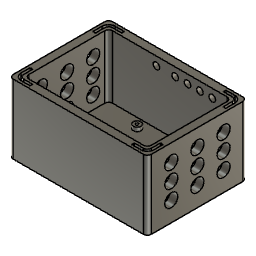
boitier_raspi (Autodesk Fusion 360 design; units mm, degrees)
Autodesk Fusion 360 part; units mm, degrees
sketch "Esquisse1" plane through (0, 0, 0) normal (0, 0, 1) x (1, 0, 0)
  line L0 (3.5419, 0) -> (103.2419, 0)
  line L1 (106.2419, 3) -> (106.2419, 73)
  line L2 (0.5419, 73) -> (0.5419, 3)
  line L3 (9.5419, 6) -> (97.2419, 6)
  line L4 (100.2419, 9) -> (100.2419, 67)
  line L5 (97.2419, 70) -> (9.5419, 70)
  line L6 (6.5419, 67) -> (6.5419, 9)
  arc A0 (100.2419, 67) -> (97.2419, 70) centre (97.2419, 67) ccw
  arc A1 (97.2419, 6) -> (100.2419, 9) centre (97.2419, 9) ccw
  arc A2 (6.5419, 9) -> (9.5419, 6) centre (9.5419, 9) ccw
  arc A3 (9.5419, 70) -> (6.5419, 67) centre (9.5419, 67) ccw
  circle A4 centre (93.7419, 62.62) radius 3
  circle A5 centre (93.7419, 62.62) radius 1.125
  circle A6 centre (93.7419, 13.62) radius 3
  circle A7 centre (93.7419, 13.62) radius 1.125
  circle A8 centre (35.7419, 13.62) radius 1.125
  circle A9 centre (35.7419, 13.62) radius 3
  circle A10 centre (35.7419, 62.62) radius 3
  circle A11 centre (35.7419, 62.62) radius 1.125
  line L7 (103.2419, 76) -> (3.5419, 76)
  arc A12 (106.2419, 73) -> (103.2419, 76) centre (103.2419, 73) ccw
  arc A13 (3.5419, 76) -> (0.5419, 73) centre (3.5419, 73) ccw
  arc A14 (0.5419, 3) -> (3.5419, 0) centre (3.5419, 3) ccw
  arc A15 (103.2419, 0) -> (106.2419, 3) centre (103.2419, 3) ccw
  line L8 (86.6419, 76) -> (86.6419, 70)
  point P0 (6.5419, 6)
  point P1 (100.2419, 6)
  point P2 (6.5419, 70)
  dimension "d5" = 6
  dimension "d6" = 6
  dimension "d7" = 3
  dimension "d8" = 3
  dimension "d9" = 3
  dimension "d10" = 3
  dimension "d34" = 6
  dimension "d37" = 2.25
  dimension "d38" = 6
  dimension "d39" = 2.25
  dimension "d40" = 6
  dimension "d41" = 2.25
  dimension "d42" = 58
  dimension "d47" = 6
  dimension "d48" = 2.25
  dimension "d52" = 6
  dimension "d77" = 64
  dimension "d80" = 6
  dimension "d85" = 7.62
  dimension "d86" = 6.5
  dimension "d88" = 7.62
  dimension "d89" = 58
  dimension "d90" = 49
  dimension "d93" = 6.5
  dimension "d94" = 49
  dimension "d101" = 3
  dimension "d102" = 3
  dimension "d103" = 3
  dimension "d104" = 3
  dimension "d105" = 7.1
  dimension "d178" = 76
  dimension "d179" = 105.7
  dimension "d223" = 29.2
  dimension "d260" = 7.38
  dimension "d263" = 13.38
  constraint horizontal L0
  constraint vertical L1
  constraint vertical L2
  constraint horizontal L3
  constraint vertical L4
  constraint horizontal L5
  constraint tangent L4 A0
  constraint tangent L5 A0
  constraint coincident P1 L3
  constraint coincident P1 L4
  constraint tangent L3 A1
  constraint tangent L4 A1
  constraint coincident P0 L3
  constraint coincident P0 L6
  constraint tangent L3 A2
  constraint tangent L6 A2
  constraint coincident P2 L5
  constraint coincident P2 L6
  constraint tangent L5 A3
  constraint tangent L6 A3
  constraint concentric A4 A5
  constraint concentric A6 A7
  constraint concentric A8 A9
  constraint concentric A10 A11
  constraint perpendicular L2 L7
  constraint tangent L7 A12
  constraint tangent L1 A12
  constraint tangent L7 A13
  constraint tangent L2 A13
  constraint tangent L0 A14
  constraint tangent L2 A14
  constraint tangent L0 A15
  constraint tangent L1 A15
  constraint coincident L7 L8.start
  constraint coincident L5 L8.end
  constraint perpendicular L5 L8
  measures "d5" distance of L0 L3
  measures "d6" distance of L1 L4
  measures "d7" radius of A0
  measures "d8" radius of A1
  measures "d9" radius of A2
  measures "d10" radius of A3
  measures "d34" diameter of A4
  measures "d37" diameter of A5
  measures "d38" diameter of A6
  measures "d39" diameter of A7
  measures "d40" diameter of A9
  measures "d41" diameter of A8
  measures "d42" distance of A6.centre A8.centre
  measures "d47" diameter of A10
  measures "d48" diameter of A11
  measures "d52" distance of L5 L7
  measures "d77" distance of L3 L5
  measures "d80" distance of L2 L6
  measures "d85" distance of L3 A6.centre
  measures "d86" distance of L4 A6.centre
  measures "d88" distance of L3 A8.centre
  measures "d89" horizontal distance of A4.centre A10.centre
  measures "d90" distance of A8.centre A10.centre
  measures "d93" distance of L4 A4.centre
  measures "d94" distance of A4.centre A6.centre
  measures "d101" radius of A12
  measures "d102" radius of A13
  measures "d103" radius of A14
  measures "d104" radius of A15
  measures "d105" distance of A4.centre L8
  measures "d178" distance of L0 L7
  measures "d179" distance of L1 L2
  measures "d223" distance of L6 A10.centre
  measures "d260" distance of L5 A10.centre
  measures "d263" distance of A4.centre L7
extrude "Extrusion1" add sketch "Esquisse1" along normal blind 5 contours L3 L4 L5 L6 A0 A1 A2 A3 | A4 | A5 | A6 | A7 | A8 | A9 | A10 | A11
extrude "Extrusion2" add sketch "Esquisse1" along normal blind 8 contours A4 | A6 | A9 | A10
extrude "Extrusion3" add sketch "Esquisse1" along normal blind 53 contours L0 L1 L2 L7 A12 A13 A14 A15
sketch "Esquisse4" plane through (0, 76, 0) normal (0, 1, 0) x (-1, 0, 0)
  line L0 (-103.2419, 0) -> (-3.5419, 0)
  line L1 (-3.5419, 0) -> (-3.5419, 53)
  line L2 (-3.5419, 53) -> (-103.2419, 53)
  line L3 (-103.2419, 53) -> (-103.2419, 0)
  line L4 (-86.7419, 0) -> (-86.7419, 10.8)
  line L5 (-81.2419, 7.3) -> (-92.2419, 7.3)
  line L6 (-92.2419, 7.3) -> (-92.2419, 14.3)
  line L7 (-92.2419, 14.3) -> (-81.2419, 14.3)
  line L8 (-81.2419, 14.3) -> (-81.2419, 7.3)
  line L9 (-81.2419, 7.3) -> (-92.2419, 14.3) construction
  line L10 (-92.2419, 7.3) -> (-81.2419, 14.3) construction
  line L11 (-91.1319, 49) -> (-39.1319, 49)
  line L12 (-39.1319, 49) -> (-39.1319, 44)
  line L13 (-39.1319, 44) -> (-91.1319, 44)
  line L14 (-91.1319, 44) -> (-91.1319, 49)
  line L15 (-106.2419, 0) -> (-106.2419, 53)
  line L16 (-83.3319, 44) -> (-88.3319, 44)
  line L17 (-88.3319, 44) -> (-88.3319, 49)
  line L18 (-88.3319, 49) -> (-83.3319, 49)
  line L19 (-83.3319, 49) -> (-83.3319, 44)
  line L20 (-83.3319, 44) -> (-88.3319, 49) construction
  line L21 (-88.3319, 44) -> (-83.3319, 49) construction
  line L22 (-73.8819, 44) -> (-78.8819, 44)
  line L23 (-78.8819, 44) -> (-78.8819, 49)
  line L24 (-78.8819, 49) -> (-73.8819, 49)
  line L25 (-73.8819, 49) -> (-73.8819, 44)
  line L26 (-73.8819, 44) -> (-78.8819, 49) construction
  line L27 (-78.8819, 44) -> (-73.8819, 49) construction
  line L28 (-64.4319, 44) -> (-69.4319, 44)
  line L29 (-69.4319, 44) -> (-69.4319, 49)
  line L30 (-69.4319, 49) -> (-64.4319, 49)
  line L31 (-64.4319, 49) -> (-64.4319, 44)
  line L32 (-64.4319, 44) -> (-69.4319, 49) construction
  line L33 (-69.4319, 44) -> (-64.4319, 49) construction
  line L34 (-54.9819, 44) -> (-59.9819, 44)
  line L35 (-59.9819, 44) -> (-59.9819, 49)
  line L36 (-59.9819, 49) -> (-54.9819, 49)
  line L37 (-54.9819, 49) -> (-54.9819, 44)
  line L38 (-54.9819, 44) -> (-59.9819, 49) construction
  line L39 (-59.9819, 44) -> (-54.9819, 49) construction
  line L40 (-40.6319, 44) -> (-45.6319, 44)
  line L41 (-45.6319, 44) -> (-45.6319, 49)
  line L42 (-45.6319, 49) -> (-40.6319, 49)
  line L43 (-40.6319, 49) -> (-40.6319, 44)
  line L44 (-40.6319, 44) -> (-45.6319, 49) construction
  line L45 (-45.6319, 44) -> (-40.6319, 49) construction
  circle A0 centre (-85.8319, 46.5) radius 2.5
  circle A1 centre (-76.3819, 46.5) radius 2.5
  circle A2 centre (-66.9319, 46.5) radius 2.5
  circle A3 centre (-57.4819, 46.5) radius 2.5
  circle A4 centre (-43.1319, 46.5) radius 2.5
  point P0 (-86.7419, 10.8)
  point P1 (-85.8319, 46.5)
  point P2 (-76.3819, 46.5)
  point P3 (-66.9319, 46.5)
  point P4 (-57.4819, 46.5)
  point P5 (-43.1319, 46.5)
  dimension "d106" = 16.5
  dimension "d107" = 10.8
  dimension "d108" = 11
  dimension "d109" = 7
  dimension "d188" = 5
  dimension "d189" = 15.11
  dimension "d190" = 52
  dimension "d225" = 5
  dimension "d226" = 5
  dimension "d227" = 5
  dimension "d228" = 5
  dimension "d229" = 5.3
  dimension "d230" = 14.75
  dimension "d231" = 5
  dimension "d232" = 5
  dimension "d233" = 5
  dimension "d234" = 5
  dimension "d235" = 24.2
  dimension "d236" = 33.65
  dimension "d237" = 5
  dimension "d238" = 5
  dimension "d239" = 48
  dimension "d264" = 4
  dimension "d265" = 4.45
  dimension "d266" = 4.45
  dimension "d267" = 4.45
  constraint coincident L0 L4.start
  constraint perpendicular L0 L4
  constraint horizontal L5
  constraint perpendicular L5 L6
  constraint parallel L5 L7
  constraint parallel L6 L8
  constraint coincident L9 P0
  constraint coincident L10 P0
  constraint coincident P0 L4.end
  constraint horizontal L11
  constraint vertical L12
  constraint horizontal L13
  constraint vertical L14
  constraint horizontal L16
  constraint perpendicular L16 L17
  constraint parallel L16 L18
  constraint parallel L17 L19
  constraint coincident L20 P1
  constraint coincident L21 P1
  constraint horizontal L22
  constraint perpendicular L22 L23
  constraint parallel L22 L24
  constraint parallel L23 L25
  constraint coincident L26 P2
  constraint coincident L27 P2
  constraint horizontal L28
  constraint perpendicular L28 L29
  constraint parallel L28 L30
  constraint parallel L29 L31
  constraint coincident L32 P3
  constraint coincident L33 P3
  constraint horizontal L34
  constraint perpendicular L34 L35
  constraint parallel L34 L36
  constraint parallel L35 L37
  constraint coincident L38 P4
  constraint coincident L39 P4
  constraint horizontal L40
  constraint perpendicular L40 L41
  constraint parallel L40 L42
  constraint parallel L41 L43
  constraint coincident L44 P5
  constraint coincident L45 P5
  constraint coincident P1 A0.centre
  constraint tangent L16 A0
  constraint coincident P2 A1.centre
  constraint tangent L22 A1
  constraint coincident P3 A2.centre
  constraint tangent L13 A2
  constraint coincident P4 A3.centre
  constraint tangent L34 A3
  constraint coincident P5 A4.centre
  constraint tangent L40 A4
  measures "d106" distance of L3 L4
  measures "d107" distance of L4.start P0
  measures "d108" distance of L6.end L7.end
  measures "d109" distance of L5.end L6.end
  measures "d188" distance of L11.end L12.end
  measures "d189" distance of L14 L15
  measures "d190" distance of L12 L14
  measures "d225" distance of L17.end L18.end
  measures "d226" distance of L16.end L17.end
  measures "d227" distance of L23.end L24.end
  measures "d228" distance of L22.end L23.end
  measures "d229" distance of L14 P1
  measures "d230" distance of L14 P2
  measures "d231" distance of L29.end L30.end
  measures "d232" distance of L28.end L29.end
  measures "d233" distance of L35.end L36.end
  measures "d234" distance of L34.end L35.end
  measures "d235" distance of L14 P3
  measures "d236" distance of L14 P4
  measures "d237" distance of L41.end L42.end
  measures "d238" distance of L40.end L41.end
  measures "d239" distance of L14 P5
  measures "d264" distance of L2 L11
  measures "d265" distance of L19 L23
  measures "d266" distance of L25 L29
  measures "d267" distance of L31 L35
extrude "Extrusion8" cut sketch "Esquisse4" against normal blind 6 contours L5 L6 L7 L8
sketch "Esquisse5" plane through (0, 0, 0) normal (0, 0, -1) x (1, 0, 0)
  arc A0 (106.2419, -3) -> (103.2419, 0) centre (103.2419, -3) ccw
  line L0 (103.2419, 0) -> (3.5419, 0)
  arc A1 (3.5419, 0) -> (0.5419, -3) centre (3.5419, -3) ccw
  line L1 (0.5419, -3) -> (0.5419, -73)
  arc A2 (0.5419, -73) -> (3.5419, -76) centre (3.5419, -73) ccw
  line L2 (3.5419, -76) -> (103.2419, -76)
  arc A3 (103.2419, -76) -> (106.2419, -73) centre (103.2419, -73) ccw
  line L3 (106.2419, -73) -> (106.2419, -3)
  line L4 (7.5419, -6) -> (17.5419, -6)
  line L5 (17.5419, -6) -> (17.5419, -16)
  line L6 (17.5419, -16) -> (7.5419, -16)
  line L7 (7.5419, -16) -> (7.5419, -6)
  line L8 (17.5419, -16) -> (12.5419, -16)
  line L9 (12.5419, -16) -> (12.5419, -11)
  line L10 (12.5419, -11) -> (17.5419, -11)
  line L11 (17.5419, -11) -> (17.5419, -16)
  line L12 (7.5419, -56) -> (17.5419, -56)
  line L13 (17.5419, -56) -> (17.5419, -66)
  line L14 (17.5419, -66) -> (7.5419, -66)
  line L15 (7.5419, -66) -> (7.5419, -56)
  line L16 (17.5419, -66) -> (12.5419, -66)
  line L17 (17.5419, -60) -> (17.5419, -66)
  line L18 (92.5419, -6) -> (82.5419, -6)
  line L19 (82.5419, -6) -> (82.5419, -16)
  line L20 (82.5419, -16) -> (92.5419, -16)
  line L21 (92.5419, -16) -> (92.5419, -6)
  line L22 (82.5419, -16) -> (87.5419, -16)
  line L23 (87.5419, -16) -> (87.5419, -11)
  line L24 (87.5419, -11) -> (82.5419, -11)
  line L25 (82.5419, -11) -> (82.5419, -16)
  line L26 (82.5419, -56) -> (92.5419, -56)
  line L27 (92.5419, -56) -> (92.5419, -66)
  line L28 (92.5419, -66) -> (82.5419, -66)
  line L29 (82.5419, -66) -> (82.5419, -56)
  line L30 (92.5419, -66) -> (87.5419, -66)
  line L31 (92.5419, -61) -> (92.5419, -66)
  line L32 (17.5419, -56) -> (12.5419, -56)
  line L33 (12.5419, -56) -> (12.5419, -61)
  line L34 (12.5419, -61) -> (17.5419, -61)
  line L35 (17.5419, -61) -> (17.5419, -56)
  line L36 (82.5419, -56) -> (87.5419, -56)
  line L37 (87.5419, -56) -> (87.5419, -61)
  line L38 (87.5419, -61) -> (82.5419, -61)
  line L39 (82.5419, -61) -> (82.5419, -56)
  dimension "d115" = 6
  dimension "d116" = 7
  dimension "d125" = 40
  dimension "d126" = 7
  dimension "d127" = 10
  dimension "d128" = 10
  dimension "d129" = 5
  dimension "d130" = 5
  dimension "d132" = 85
  dimension "d133" = 6
  dimension "d134" = 10
  dimension "d135" = 10
  dimension "d137" = 5
  dimension "d138" = 10
  dimension "d139" = 10
  dimension "d140" = 5
  dimension "d141" = 5
  dimension "d142" = 40
  dimension "d143" = 10
  dimension "d144" = 5
  dimension "d145" = 10
  dimension "d146" = 85
  dimension "d147" = 5
  dimension "d148" = 5
  dimension "d149" = 5
  dimension "d150" = 5
  constraint horizontal L4
  constraint vertical L5
  constraint horizontal L6
  constraint vertical L7
  constraint horizontal L8
  constraint vertical L9
  constraint horizontal L10
  constraint vertical L11
  constraint horizontal L12
  constraint vertical L13
  constraint horizontal L14
  constraint vertical L15
  constraint horizontal L16
  constraint vertical L17
  constraint horizontal L18
  constraint vertical L19
  constraint horizontal L20
  constraint vertical L21
  constraint horizontal L22
  constraint vertical L23
  constraint horizontal L24
  constraint vertical L25
  constraint horizontal L26
  constraint vertical L27
  constraint horizontal L28
  constraint vertical L29
  constraint horizontal L30
  constraint vertical L31
  constraint horizontal L32
  constraint vertical L33
  constraint horizontal L34
  constraint vertical L35
  constraint horizontal L36
  constraint vertical L37
  constraint horizontal L38
  constraint vertical L39
  measures "d115" distance of L0 L4
  measures "d116" distance of L1 L7
  measures "d125" distance of L6 L12
  measures "d126" distance of L1 L15
  measures "d127" distance of L18.start L18.end
  measures "d128" distance of L18.start L20.end
  measures "d129" distance of L19.end L22.end
  measures "d130" distance of L19.end L24.end
  measures "d132" distance of L7 L21
  measures "d133" distance of L0 L18
  measures "d134" distance of L5.end L6.end
  measures "d135" distance of L12.start L12.end
  measures "d137" distance of L9.end L10.end
  measures "d138" distance of L26.start L26.end
  measures "d139" distance of L26.start L28.end
  measures "d140" distance of L27.end L30.end
  measures "d141" distance of L27.end L31.start
  measures "d142" distance of L20 L26
  measures "d143" distance of L4.end L5.end
  measures "d144" distance of L8.end L9.end
  measures "d145" distance of L12.end L13.end
  measures "d146" distance of L15 L27
  measures "d147" distance of L12.end L32.end
  measures "d148" distance of L12.end L34.end
  measures "d149" distance of L26.start L36.end
  measures "d150" distance of L26.start L38.end
extrude "Extrusion9" cut sketch "Esquisse5" against normal blind 3 contours L4 L5 L6 L7 L9 L10 | L12 L13 L14 L15 L16 L17 L33 L34 | L18 L19 L20 L21 L23 L24 | L26 L27 L28 L29 L30 L31 L37 L38
sketch "Esquisse6" plane through (0, 0, 53) normal (0, 0, 1) x (-1, 0, 0)
  arc A0 (-9.5419, -70) -> (-6.5419, -67) centre (-9.5419, -67) ccw
  line L0 (-9.5419, -70) -> (-97.2419, -70)
  arc A1 (-100.2419, -67) -> (-97.2419, -70) centre (-97.2419, -67) ccw
  line L1 (-100.2419, -67) -> (-100.2419, -9)
  arc A2 (-97.2419, -6) -> (-100.2419, -9) centre (-97.2419, -9) ccw
  line L2 (-97.2419, -6) -> (-9.5419, -6)
  arc A3 (-6.5419, -9) -> (-9.5419, -6) centre (-9.5419, -9) ccw
  line L3 (-6.5419, -9) -> (-6.5419, -67)
  arc A4 (-103.2419, 0) -> (-106.2419, -3) centre (-103.2419, -3) ccw
  line L4 (-106.2419, -3) -> (-106.2419, -73)
  arc A5 (-106.2419, -73) -> (-103.2419, -76) centre (-103.2419, -73) ccw
  line L5 (-103.2419, -76) -> (-3.5419, -76)
  arc A6 (-3.5419, -76) -> (-0.5419, -73) centre (-3.5419, -73) ccw
  line L6 (-0.5419, -73) -> (-0.5419, -3)
  arc A7 (-0.5419, -3) -> (-3.5419, 0) centre (-3.5419, -3) ccw
  line L7 (-3.5419, 0) -> (-103.2419, 0)
  line L8 (-103.2419, -76) -> (-3.5419, -76)
  line L9 (-0.5419, -73) -> (-0.5419, -3)
  line L10 (-106.2419, -3) -> (-106.2419, -73)
  line L11 (-3.5419, 0) -> (-103.2419, 0)
  line L12 (-14.5419, -74) -> (-7.5419, -74)
  line L13 (-2.5419, -69) -> (-2.5419, -62)
  arc A8 (-7.5419, -74) -> (-2.5419, -69) centre (-7.5419, -69) ccw
  line L14 (-14.5419, -72) -> (-7.5419, -72)
  arc A9 (-7.5419, -72) -> (-4.5419, -69) centre (-7.5419, -69) ccw
  line L15 (-4.5419, -69) -> (-4.5419, -62)
  line L16 (-14.5419, -74) -> (-14.5419, -72)
  line L17 (-4.5419, -62) -> (-2.5419, -62)
  line L18 (-92.2419, -74) -> (-99.2419, -74)
  line L19 (-104.2419, -69) -> (-104.2419, -62)
  arc A10 (-104.2419, -69) -> (-99.2419, -74) centre (-99.2419, -69) ccw
  line L20 (-92.2419, -72) -> (-99.2419, -72)
  arc A11 (-102.2419, -69) -> (-99.2419, -72) centre (-99.2419, -69) ccw
  line L21 (-102.2419, -69) -> (-102.2419, -62)
  line L22 (-92.2419, -74) -> (-92.2419, -72)
  line L23 (-102.2419, -62) -> (-104.2419, -62)
  line L24 (-104.2419, -14) -> (-104.2419, -7)
  line L25 (-99.2419, -2) -> (-92.2419, -2)
  arc A12 (-99.2419, -2) -> (-104.2419, -7) centre (-99.2419, -7) ccw
  line L26 (-92.2419, -2) -> (-92.2419, -4)
  line L27 (-102.2419, -14) -> (-104.2419, -14)
  line L28 (-102.2419, -14) -> (-102.2419, -7)
  arc A13 (-99.2419, -4) -> (-102.2419, -7) centre (-99.2419, -7) ccw
  line L29 (-99.2419, -4) -> (-92.2419, -4)
  line L30 (-2.5419, -14) -> (-2.5419, -7)
  line L31 (-7.5419, -2) -> (-14.5419, -2)
  arc A14 (-2.5419, -7) -> (-7.5419, -2) centre (-7.5419, -7) ccw
  line L32 (-4.5419, -14) -> (-4.5419, -7)
  arc A15 (-4.5419, -7) -> (-7.5419, -4) centre (-7.5419, -7) ccw
  line L33 (-7.5419, -4) -> (-14.5419, -4)
  line L34 (-2.5419, -14) -> (-4.5419, -14)
  line L35 (-14.5419, -4) -> (-14.5419, -2)
  dimension "d277" = 5
  dimension "d278" = -2
  dimension "d279" = 2
  dimension "d280" = 2
  dimension "d281" = 12
  dimension "d282" = 12
  dimension "d283" = 5
  dimension "d284" = -2
  dimension "d285" = 12
  dimension "d286" = 12
  dimension "d287" = 5
  dimension "d288" = 2
  dimension "d289" = 2
  dimension "d290" = 2
  dimension "d291" = 2
  dimension "d292" = 2
  dimension "d293" = 12
  dimension "d294" = 12
  dimension "d295" = 2
  dimension "d296" = 2
  dimension "d297" = 5
  dimension "d298" = -2
  dimension "d299" = 12
  dimension "d300" = 12
  constraint horizontal L12
  constraint perpendicular L12 L13
  constraint tangent L12 A8
  constraint tangent L13 A8
  constraint perpendicular L13 L17
  constraint parallel L8 L18
  constraint perpendicular L8 L19
  constraint tangent L18 A10
  constraint tangent L19 A10
  constraint perpendicular L19 L23
  constraint parallel L4 L24
  constraint perpendicular L24 L25
  constraint tangent L24 A12
  constraint tangent L25 A12
  constraint perpendicular L25 L26
  constraint perpendicular L24 L27
  constraint vertical L30
  constraint perpendicular L30 L31
  constraint tangent L30 A14
  constraint tangent L31 A14
  constraint perpendicular L31 L35
  measures "d277" radius of A8
  measures "d279" distance of L8 L12
  measures "d280" distance of L9 L13
  measures "d281" distance of L12 L17
  measures "d282" distance of L13 L16
  measures "d283" radius of A10
  measures "d285" distance of L18 L23
  measures "d286" distance of L19 L22
  measures "d287" radius of A12
  measures "d288" distance of L10 L19
  measures "d289" distance of L8 L18
  measures "d290" distance of L10 L24
  measures "d291" distance of L11 L25
  measures "d293" distance of L25 L27
  measures "d294" distance of L24 L26
  measures "d295" distance of L11 L31
  measures "d296" distance of L9 L30
  measures "d297" radius of A14
  measures "d299" distance of L31 L34
  measures "d300" distance of L30 L35
extrude "Extrusion18" cut sketch "Esquisse6" against normal blind 6 contours L12 L13 A8 L14 A9 L15 L16 L17 | L18 L19 A10 L20 A11 L21 L22 L23 | L24 L25 A12 L26 L27 L28 A13 L29 | L30 L31 A14 L32 A15 L33 L34 L35
sketch "Esquisse7" plane through (0, 0, 0) normal (0, -1, 0) x (1, 0, 0)
  line L0 (3.5419, 0) -> (103.2419, 0)
  line L1 (103.2419, 0) -> (103.2419, 53)
  line L2 (103.2419, 53) -> (3.5419, 53)
  line L3 (3.5419, 53) -> (3.5419, 0)
  line L4 (35.4919, 44.63) -> (21.1919, 44.63)
  line L5 (21.1919, 44.63) -> (21.1919, 41.93)
  line L6 (21.1919, 41.93) -> (35.4919, 41.93)
  line L7 (35.4919, 41.93) -> (35.4919, 44.63)
  line L8 (35.4919, 44.63) -> (21.1919, 41.93) construction
  line L9 (21.1919, 44.63) -> (35.4919, 41.93) construction
  line L10 (106.2419, 0) -> (106.2419, 53)
  line L11 (3.5419, 0) -> (103.2419, 0)
  point P0 (28.3419, 43.28)
  dimension "d183" = 14.3
  dimension "d184" = 2.7
  dimension "d253" = 77.9
  dimension "d254" = 43.28
  constraint horizontal L4
  constraint perpendicular L4 L5
  constraint parallel L4 L6
  constraint parallel L5 L7
  constraint coincident L8 P0
  constraint coincident L9 P0
  measures "d183" distance of L5.end L6.end
  measures "d184" distance of L4.end L5.end
  measures "d253" distance of P0 L10
  measures "d254" distance of P0 L11
extrude "Extrusion13" cut 4 faces at (93.6585, 62.6769, 5) (93.7699, 14.4164, 5) (35.4196, 13.2423, 5) (35.0663, 62.8029, 5) along direction (0, 0, -1) blind 3
sketch "Esquisse8" plane through (106.2419, 0, 0) normal (1, 0, 0) x (0, 1, 0)
  line L0 (3, 0) -> (73, 0)
  line L1 (73, 0) -> (73, 53)
  line L2 (73, 53) -> (3, 53)
  line L3 (3, 53) -> (3, 0)
  circle A0 centre (18.25, 40) radius 5
  circle A1 centre (38.25, 40) radius 5
  circle A2 centre (58.25, 40) radius 5
  circle A3 centre (18.25, 27.5) radius 5
  circle A4 centre (38.25, 27.5) radius 5
  circle A5 centre (58.25, 27.5) radius 5
  circle A6 centre (18.25, 15) radius 5
  circle A7 centre (38.25, 15) radius 5
  circle A8 centre (58.25, 15) radius 5
  line L4 (0, 0) -> (0, 53)
  line L5 (76, 0) -> (76, 53)
  line L6 (3, 53) -> (73, 53)
  line L7 (3, 0) -> (73, 0)
  dimension "d242" = 10
  dimension "d245" = 40
  dimension "d246" = -25
  dimension "d247" = 18.25
  dimension "d248" = 17.75
  dimension "d249" = 13
  dimension "d250" = 15
  measures "d242" diameter of A0
  measures "d247" distance of A0.centre L4
  measures "d248" distance of A2.centre L5
  measures "d249" distance of A1.centre L6
  measures "d250" distance of A7.centre L7
extrude "Extrusion16" cut sketch "Esquisse8" against normal blind 150 contours A0 | A1 | A2 | A3 | A4 | A5 | A6 | A7 | A8
extrude "Extrusion17" cut sketch "Esquisse4" against normal blind 6 contours A0 | A1 | A2 | A3 | A4
equation "d37 = d48"
equation "d39 = d48"
equation "d41 = d48"
equation "d85 = d88"
equation "d88 = 3.5 mm + 4.12 mm"
equation "d107 = 8 mm + 2.8 mm"
equation "d146 = d132"
equation "d189 = 9.11 mm + 6 mm"
equation "d223 = 23.5 mm + 5.7 mm"
equation "d279 = d280"
equation "d282 = d281"
equation "d284 = d278"
equation "d285 = d281"
equation "d286 = d285"
